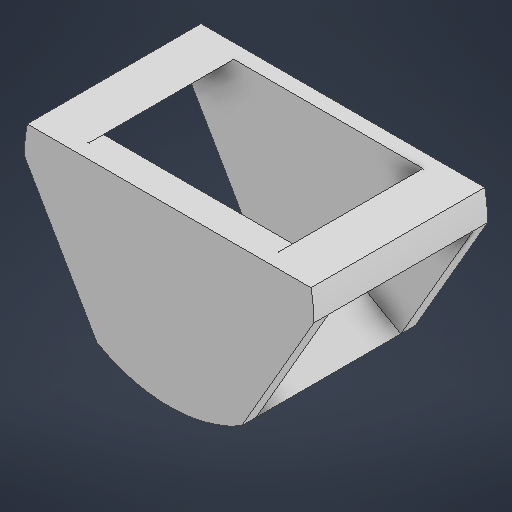
# Autodesk Inventor part: BodyFoldedSide1
Saved by Autodesk Inventor 2026.2 (Build 302298000, 298)
## iProperties
Created: 2025-11-02
Part Number: BodyFoldedSide1
Material: Generic
Document SubType Name: Modeling
Designer: kubek
Density: 1 g/cm^3
Appearance: Default
Author: kubek
Autodesk Inventor part; units mm, degrees
ref_plane "YZ Plane" through (0, 0, 0) normal (1, 0, 0) x (0, 1, 0)
ref_plane "XZ Plane" through (0, 0, 0) normal (0, 1, 0) x (-1, 0, 0)
sketch "Sketch9" plane through (0, 0, 0) normal (0, 0, 1) x (1, 0, 0)
  line L0 (5, 0) -> (2.5, -4.3301)
  line L1 (2.5, -4.3301) -> (-2.5, -4.3301)
  line L2 (-2.5, -4.3301) -> (-5, 0)
  line L3 (-5, 0) -> (-2.5, 4.3301)
  line L4 (-2.5, 4.3301) -> (2.5, 4.3301)
  line L5 (2.5, 4.3301) -> (5, 0)
  line L6 (2.5, 4.3301) -> (2.5, 2.3301)
  line L7 (2.5, 2.3301) -> (-2.5, 2.3301)
  line L8 (-2.5, 2.3301) -> (-2.5, 4.3301)
  line L9 (-2.5, -4.3301) -> (-5, 0)
  line L10 (-0.7679, -3.3301) -> (-2.5, -4.3301)
  line L11 (-3.2679, 1) -> (-0.7679, -3.3301)
  line L12 (-5, 0) -> (-3.2679, 1)
  line L13 (5, 0) -> (2.5, -4.3301)
  line L14 (3.2679, 1) -> (5, 0)
  line L15 (0.7679, -3.3301) -> (3.2679, 1)
  line L16 (2.5, -4.3301) -> (0.7679, -3.3301)
  point P0 (0, 0)
  point P1 (0, 0)
  point P2 (-5, 0)
  dimension "d62" = 5
  dimension "d63" = 2
  dimension "d66" = 360
  constraints: 34 end point, 1 coincident, 1 parallel, 41 other
  measures "d62" distance of L3.end L4.end
  measures "d63" distance of L6.start L6.end
extrude "Extrusion9" add sketch "Sketch9" against normal blind 0.5 contours L14 L15 L16 L1 L10 L11 L12 L3 L8 L7 L6 L5
sketch "Sketch11" plane through (0, 0, -0.5) normal (0, 0, -1) x (-1, 0, 0)
  line L0 (2.5, 2.3301) -> (-2.5, 2.3301) projected
  line L1 (-2.5, 2.3301) -> (-2.5, 4.3301) projected
  line L2 (-2.5, 2.3301) -> (-2.5, 4.3301)
  line L3 (-5, 0) -> (-2.5, 4.3301) projected
  line L4 (-2.5, 4.3301) -> (-5, 0)
  line L5 (-3.2679, 1) -> (-0.7679, -3.3301) projected
  line L6 (-5, 0) -> (-3.2679, 1)
  line L7 (-3.2679, 1) -> (-2.5, 2.3301)
  line L8 (2.5, 4.3301) -> (2.5, 2.3301) projected
  line L9 (2.5, 4.3301) -> (2.5, 2.3301)
  line L10 (2.5, 2.3301) -> (3.2679, 1)
  line L11 (3.2679, 1) -> (5, 0)
  line L12 (5, 0) -> (2.5, 4.3301)
  line L13 (-0.7679, -3.3301) -> (-2.5, -4.3301)
  line L14 (2.5, -4.3301) -> (0.7679, -3.3301) projected
  line L15 (-2.5, -4.3301) -> (2.5, -4.3301)
  line L16 (2.5, -4.3301) -> (0.7679, -3.3301)
  line L17 (0.7679, -3.3301) -> (-0.7679, -3.3301)
  point P0 (0, 0)
  constraints: 24 end point, 5 perpendicular, 3 parallel, 2 collinear, 2 vertical, 1 point on line
extrude "Extrusion10" add sketch "Sketch11" along normal blind 4.5
sketch "Sketch12" plane through (0, 0, 0) normal (0, 0, 1) x (1, 0, 0)
  line L0 (3.2679, 1) -> (5, 0) projected
  line L1 (-2.5, 4.3301) -> (-5, 0)
  line L2 (-2.5, -4.3301) -> (2.5, -4.3301)
  line L3 (2.5, 4.3301) -> (2.5, 2.3301) projected
  line L4 (5, 0) -> (2.5, 4.3301)
  arc A0 (-2.5, 4.3301) -> (-5, 0) centre (0, 0) ccw
  arc A1 (-2.5, -4.3301) -> (2.5, -4.3301) centre (0, 0) ccw
  arc A2 (5, 0) -> (2.5, 4.3301) centre (0, 0) ccw
  constraints: 7 point on circle, 6 end point, 3 centre point, 1 coincident, 1 horizontal
extrude "Extrusion11" add sketch "Sketch12" against normal blind 5
extrude "Extrusion12" add sketch "Sketch9" along normal blind 0.5
extrude "Extrusion13" add sketch "Sketch12" along normal blind 0.5
ref_plane "Work Plane1" through (3.2679, 1, -5) normal (0, 1, 0) x (-1, 0, 0)
split "Split1" plane through (3.2679, 1, -5) removes the side toward (0, 1, 0)
sketch "Sketch14" plane through (0, 0, -5) normal (0, 0, -1) x (-1, 0, 0)
  arc A0 (-2.5, -4.3301) -> (2.5, -4.3301) centre (0, 0) ccw projected
  line L0 (5, 0) -> (2.5, -4.3301) projected
  line L1 (5, 0) -> (2.5, -4.3301)
  line L2 (-2.5, -4.3301) -> (-5, 0) projected
  line L3 (-2.5, -4.3301) -> (-5, 0)
  line L4 (4.899, 1) -> (-4.899, 1)
  line L5 (3.2679, 1) -> (-3.2679, 1) projected
  arc A1 (5, 0) -> (4.899, 1) centre (0, 0) ccw
  arc A2 (-4.899, 1) -> (-5, 0) centre (0, 0) ccw
  arc A3 (-2.5, -4.3301) -> (2.5, -4.3301) centre (0, 0) ccw
  constraints: 6 end point, 6 point on circle, 3 centre point, 2 collinear, 1 coincident
extrude "Extrusion14" add sketch "Sketch14" along normal blind 0.5
body "Solid3"
